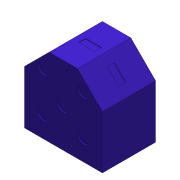
# Autodesk Inventor part: bodyy
Saved by Autodesk Inventor 2018 (Build 220112000, 112)
## iProperties
Created: 2019-12-19
Part Number: bodyy
Material: Generic
Document SubType Name: Modeling
Designer: Ibnu
Density: 1 g/cm^3
Appearance: Default
Mass: 6505.68 g
Surface Area: 2089.8 cm^2
Volume: 6505.68 cm^3
Author: Ibnu
Autodesk Inventor part; units mm, degrees
ref_plane "YZ Plane" through (0, 0, 0) normal (1, 0, 0) x (0, 1, 0)
ref_plane "XZ Plane" through (0, 0, 0) normal (0, 1, 0) x (-1, 0, 0)
ref_plane "XY Plane" through (0, 0, 0) normal (0, 0, 1) x (1, 0, 0)
sketch "Sketch1" plane through (0, 0, 0) normal (0, 1, 0) x (-1, 0, 0)
  line L0 (110, -110) -> (-110, -110)
  line L1 (-110, -110) -> (-110, 110)
  line L2 (-110, 110) -> (110, 110)
  line L3 (110, 110) -> (110, -110)
  dimension "d2" = 220
  dimension "d3" = 220
  constraints: 8 end point, 2 parallel, 1 horizontal, 1 perpendicular
  measures "d2" distance of L1.end L2.end
  measures "d3" distance of L0.end L1.end
extrude "Extrusion1" add sketch "Sketch1" along normal blind 150
sketch "Sketch2" plane through (-110, 0, 110) normal (0, 0, 1) x (1, 0, 0)
  line L0 (220, 150) -> (0, 150) projected
  line L1 (0, 0) -> (220, 0) projected
  line L2 (0, 0) -> (0, 150) projected
  line L3 (87.5, 85) -> (132.5, 85)
  line L4 (132.5, 85) -> (132.5, 65)
  line L5 (132.5, 65) -> (87.5, 65)
  line L6 (87.5, 65) -> (87.5, 85)
  line L7 (87.5, 85) -> (132.5, 65) construction
  line L8 (132.5, 85) -> (87.5, 65) construction
  point P0 (110, 0)
  point P1 (110, 75)
  dimension "d6" = 45
  dimension "d7" = 20
  constraints: 12 end point, 2 midpoint, 2 parallel, 1 horizontal, 1 perpendicular
  measures "d6" distance of L4.end L5.end
  measures "d7" distance of L3.end L4.end
extrude "Extrusion2" cut sketch "Sketch2" against normal blind 1.5
chamfer "Chamfer1" distance 70 angle 45 2 edges at (110, 75, 110) (-110, 75, 110)
sketch "Sketch3" plane through (40, 0, 110) normal (0.7071, 0, 0.7071) x (0.7071, 0, -0.7071)
  line L0 (26.9975, 65) -> (71.9975, 65)
  line L1 (71.9975, 65) -> (71.9975, 85)
  line L2 (71.9975, 85) -> (26.9975, 85)
  line L3 (26.9975, 85) -> (26.9975, 65)
  line L4 (26.9975, 65) -> (71.9975, 85) construction
  line L5 (71.9975, 65) -> (26.9975, 85) construction
  point P0 (49.4975, 75)
  dimension "d13" = 45
  dimension "d14" = 20
  constraints: 12 end point, 2 midpoint, 2 parallel, 1 horizontal, 1 perpendicular
  measures "d13" distance of L2.end L1.end
  measures "d14" distance of L1.end L0.end
extrude "Extrusion3" cut sketch "Sketch3" against normal blind 1.5
sketch "Sketch4" plane through (-110, 0, 40) normal (-0.7071, 0, 0.7071) x (0.7071, 0, 0.7071)
  line L0 (26.9975, 85) -> (71.9975, 85)
  line L1 (71.9975, 85) -> (71.9975, 65)
  line L2 (71.9975, 65) -> (26.9975, 65)
  line L3 (26.9975, 65) -> (26.9975, 85)
  line L4 (26.9975, 85) -> (71.9975, 65) construction
  line L5 (71.9975, 85) -> (26.9975, 65) construction
  point P0 (49.4975, 75)
  dimension "d17" = 45
  dimension "d18" = 20
  constraints: 12 end point, 2 midpoint, 2 parallel, 1 horizontal, 1 perpendicular
  measures "d17" distance of L1.end L2.end
  measures "d18" distance of L0.end L1.end
extrude "Extrusion4" cut sketch "Sketch4" against normal blind 1.5
sketch "Sketch5" plane through (0, 0, 0) normal (0, -1, 0) x (1, 0, 0)
  circle A0 centre (-55.0452, 64.279) radius 18
  circle A1 centre (0, 0) radius 18
  circle A2 centre (0, 0) radius 18
  circle A3 centre (57.3798, 63.8751) radius 18
  circle A4 centre (-55.4491, -48.146) radius 18
  circle A5 centre (56.9759, -48.5499) radius 18
  constraints: 6 centre point
extrude "Extrusion7" cut sketch "Sketch5" against normal blind 3
body "Solid1"
